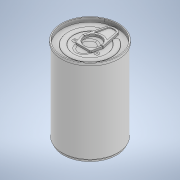
# Autodesk Inventor part: SoupCan
Saved by Autodesk Inventor 2020 (Build 240168000, 168)
## iProperties
Created: 2023-01-12
Part Number: SoupCan
Material: Generic
Document SubType Name: Modeling
Designer: legoo
Density: 1 g/cm^3
Appearance: Default
Author: legoo
Autodesk Inventor part; units mm, degrees
ref_plane "XZ Plane" through (0, 0, 0) normal (0, 1, 0) x (-1, 0, 0)
ref_plane "XY Plane" through (0, 0, 0) normal (0, 0, 1) x (1, 0, 0)
sketch "Sketch1" plane through (0, 0, 0) normal (0, 0, 1) x (1, 0, 0)
  line L0 (32.75, 4.0593) -> (32.75, 99.4351)
  line L1 (32.35, 97.4351) -> (0, 97.4351)
  line L2 (0, 97.4351) -> (0, 3.7133)
  line L3 (32.75, 99.4351) -> (33.55, 99.4351)
  line L4 (33.55, 99.4351) -> (33.55, 102.2351)
  line L5 (33.55, 102.2351) -> (32.35, 102.2351)
  line L6 (32.35, 102.2351) -> (32.35, 97.4351)
  line L7 (15, 3.7133) -> (0, 3.7133)
  arc A0 (15, 3.7133) -> (19.7851, 2.9089) centre (17.6851, 5.0514) ccw
  arc A1 (22.5851, 2.9089) -> (26.5659, 2.7142) centre (24.6851, 5.0514) ccw
  arc A2 (22.5851, 2.9089) -> (19.7851, 2.9089) centre (21.1851, 1.4807) ccw
  arc A3 (29.3384, 2.4576) -> (26.5659, 2.7142) centre (27.8198, 1.1561) ccw
  arc A4 (31.8792, 2.7098) -> (32.75, 4.0593) centre (30.8031, 4.3599) ccw
  arc A5 (31.2467, 0.7007) -> (31.8792, 2.7098) centre (28.3022, 2.7319) ccw
  arc A6 (29.9974, 0.7007) -> (31.2467, 0.7007) centre (30.622, 1.3024) ccw
  line L8 (29.3384, 2.4576) -> (29.9974, 0.7007)
  point P0 (0, 0)
  point P1 (30.622, 0.4351)
  dimension "d0" = 1.2
  dimension "d1" = 0.8
  dimension "d2" = 2.8
  dimension "d3" = 4.8
  dimension "d5" = 32.75
  dimension "d7" = 2
  dimension "d8" = 3
  dimension "d10" = 3
  dimension "d11" = 7
  dimension "d13" = 0
  dimension "d14" = 2
  dimension "d15" = 0
  dimension "d16" = 15
  dimension "d18" = 101.8
  dimension "d19" = 0.4351
  constraints: 18 end point, 16 point on circle, 7 centre point, 3 parallel, 3 tangent, 1 horizontal, 1 perpendicular
  measures "d0" distance of L4.end L5.end
  measures "d1" distance between parallel lines of L4 L0
  measures "d2" distance of L3.end L4.end
  measures "d3" distance between parallel lines of L1 L5
  measures "d5" distance between parallel lines of L2 L0
  measures "d7" radius of A2
  measures "d8" radius of A0
  measures "d10" radius of A1
  measures "d11" distance of A1.centre A0.centre
  measures "d13" vertical distance of A0.centre A1.centre
  measures "d14" radius of A3
  measures "d15" distance from line of point (0, 0) L2
  measures "d16" distance of L7.start L2.end
  measures "d18" distance from line of L5 point (30.622, 0.435)
  measures "d19" vertical distance of point (0, 0) point (30.622, 0.435)
revolve "Revolution1" add sketch "Sketch1" angle 360 about axis through (0, 97.4351, 0) along (0, -1, 0)
sketch "Sketch2" plane through (0, 97.4351, 0) normal (0, 1, 0) x (1, 0, 0)
  arc A0 (-12.675, 21.9537) -> (12.675, 21.9537) centre (0, 0) ccw
  arc A1 (-9.675, 16.7576) -> (9.675, 16.7576) centre (0, 0) ccw
  line L0 (0, 0) -> (-14.6692, 25.4078) construction
  line L1 (0, 0) -> (14.3618, 24.8753) construction
  circle A2 centre (0, 0) radius 32.35 construction
  circle A3 centre (0, 0) radius 22.35 construction
  arc A4 (-9.675, 16.7576) -> (-12.675, 21.9537) centre (-11.175, 19.3557) ccw
  arc A5 (12.675, 21.9537) -> (9.675, 16.7576) centre (11.175, 19.3557) ccw
  line L2 (0, 0) -> (0, 29.3384) construction
  circle A6 centre (0, 0) radius 29.3384 construction
  dimension "d20" = 6
  dimension "d21" = 7
  dimension "d22" = 3
  dimension "d23" = 60
  dimension "d48" = 30
  dimension "d53" = 0
  dimension "d54" = 0
  constraints: 10 point on circle, 6 end point, 5 centre point, 4 point on line, 3 coincident, 1 vertical, 2 other
  measures "d20" radial gap between concentric circles of A1 A0
  measures "d21" radial gap between concentric circles of A0 A2
  measures "d22" radial gap between concentric circles of A3 A0
  measures "d23" angle of L1 L0
  measures "d48" angle of L1 L2
  measures "d53" distance of point (0, 0) L1.start
  measures "d54" distance of point (0, 0) L1.start
extrude "Extrusion1" add sketch "Sketch2" along normal blind 0.25
chamfer "Chamfer1" distance 0.25 angle 45 4 edges at (0, 97.4351, 25.35) (-8.5769, 97.4351, -20.8557) (0, 97.4351, 19.35) (8.5769, 97.4351, -20.8557)
sketch "Sketch3" plane through (0, 97.4351, 0) normal (0, 1, 0) x (1, 0, 0)
  ellipse E0 centre (0, -4.1) end of major axis (0, 5.9) minor radius 7.5
  arc A0 (-9.55, 16.5411) -> (9.55, 16.5411) centre (0, 0) ccw construction
  point P0 (0, 0)
  point P1 (0, -19.1)
  point P2 (0, -14.1)
  dimension "d29" = 10
  dimension "d30" = 7.5
  dimension "d31" = 5
  constraints: 1 point on circle, 1 vertical alignment, 2 other
  measures "d31" distance of point (0, -14.1) point (0, -19.1)
extrude "Extrusion2" cut sketch "Sketch3" against normal blind 0.6
chamfer "Chamfer2" distance 0.6 distance2 2.5 1 edges at (0, 97.4351, 14.1) measured on face at (-7.3349, 97.0351, 6.1869)
sketch "Sketch4" plane through (0, 97.4351, 0) normal (0, 1, 0) x (1, 0, 0)
  circle A0 centre (-13, -4.85) radius 2.5
  circle A1 centre (13, -4.85) radius 2.5
  arc A2 (-9.675, 16.7576) -> (9.675, 16.7576) centre (0, 0) ccw construction
  point P0 (0, 0)
  point P1 (0, -19.35)
  dimension "d37" = 5
  dimension "d38" = 5
  dimension "d39" = 14.5
  dimension "d40" = 14.5
  dimension "d41" = 13
  dimension "d42" = 13
  constraints: 2 centre point, 1 point on circle
  measures "d37" diameter of A1
  measures "d38" diameter of A0
  measures "d39" vertical distance of point (0, -19.35) A0.centre
  measures "d40" vertical distance of point (0, -19.35) A1.centre
  measures "d41" horizontal distance of A0.centre point (0, 0)
  measures "d42" horizontal distance of point (0, 0) A1.centre
extrude "Extrusion3" add sketch "Sketch4" along normal blind 0.6
fillet "Fillet1" radius 2.5 2 edges at (10.5, 98.0351, 4.85) (-15.5, 98.0351, 4.85)
sketch "Sketch5" plane through (0, 97.4351, 0) normal (0, 1, 0) x (1, 0, 0)
  ellipse E0 centre (0, 25.85) end of major axis (-6.85, 25.85) minor radius 4 (6.85, 25.85) -> (-6.85, 25.85) ccw
  circle A0 centre (0, 0) radius 32.35 construction
  line L0 (6.85, 25.85) -> (11.7977, 3.6347)
  line L1 (-6.85, 25.85) -> (-11.7977, 3.6347)
  line L2 (11.7899, 3.1673) -> (9.0436, -7.4689)
  line L3 (-11.7899, 3.1673) -> (-9.0436, -7.4689)
  line L4 (-8.0754, -8.2189) -> (8.0754, -8.2189)
  arc A1 (-9.0436, -7.4689) -> (-8.0754, -8.2189) centre (-8.0754, -7.2189) ccw
  arc A2 (8.0754, -8.2189) -> (9.0436, -7.4689) centre (8.0754, -7.2189) ccw
  arc A3 (11.7899, 3.1673) -> (11.7977, 3.6347) centre (10.8217, 3.4173) ccw
  arc A4 (-11.7977, 3.6347) -> (-11.7899, 3.1673) centre (-10.8217, 3.4173) ccw
  point P0 (0, 32.35)
  point P1 (0, 29.85)
  point P2 (0, 29.85)
  point P3 (11.85, 3.4001)
  point P4 (-11.85, 3.4001)
  point P5 (8.85, -8.2189)
  point P6 (-8.85, -8.2189)
  dimension "d46" = 6.85
  dimension "d47" = 4
  dimension "d49" = 0
  dimension "d50" = 2.5
  dimension "d51" = 0
  dimension "d52" = 0
  dimension "d57" = 5
  dimension "d59" = 23
  dimension "d60" = 23
  dimension "d61" = 5
  dimension "d62" = 3
  dimension "d63" = 3
  dimension "d64" = 12
  dimension "d65" = 12
  dimension "d68" = 0
  dimension "d69" = 0
  dimension "d70" = 1
  constraints: 10 end point, 8 point on circle, 8 point on line, 8 tangent, 4 centre point, 3 equal radius, 1 coincident, 1 vertical alignment, 6 other
  measures "d49" horizontal distance of point (0, 0) point (0, 25.85)
  measures "d50" distance of point (0, 32.35) point (0, 29.85)
  measures "d51" horizontal distance of point (0, 0) point (0, 29.85)
  measures "d52" horizontal distance of point (0, 0) point (0, 32.35)
  measures "d57" horizontal distance of point (11.85, 3.4) L0.start
  measures "d59" distance of L0.start point (11.85, 3.4)
  measures "d60" distance of L1.start point (-11.85, 3.4)
  measures "d61" horizontal distance of point (-11.85, 3.4) L1.start
  measures "d62" horizontal distance of point (8.85, -8.219) point (11.85, 3.4)
  measures "d63" horizontal distance of point (-11.85, 3.4) point (-8.85, -8.219)
  measures "d64" distance of point (11.85, 3.4) point (8.85, -8.219)
  measures "d65" distance of point (-11.85, 3.4) point (-8.85, -8.219)
  measures "d68" vertical distance of point (0, 25.85) L0.start
  measures "d69" vertical distance of point (0, 25.85) L1.start
  measures "d70" radius of A1
extrude "Extrusion4" add sketch "Sketch5" along normal blind 2.6
ref_plane "Work Plane1" through (-12.7, 0, 0) normal (1, 0, 0) x (0, 1, 0)
sketch "Sketch6" plane through (-12.7, 0, 0) normal (1, 0, 0) x (0, 1, 0)
  line L0 (99.4351, 32.75) -> (99.4351, -32.75) projected
  line L1 (99.4351, -29.7539) -> (100.0351, -3.6347)
  line L2 (100.0351, -3.6347) -> (100.0351, -3.1673) projected
  line L3 (100.0351, -3.6347) -> (100.0351, -3.1673)
  line L4 (100.0351, -3.1673) -> (99.4351, 8.2189)
  line L5 (97.4351, 8.2189) -> (100.0351, 8.2189) projected
  line L6 (99.4351, 8.2189) -> (104.5755, 8.3468)
  line L7 (104.5755, 8.3468) -> (104.5755, -29.7539)
  line L8 (104.5755, -29.7539) -> (99.4351, -29.7539)
  point P0 (0, 0)
  constraints: 12 end point, 2 point on line, 1 perpendicular, 1 vertical
extrude "Extrusion5" cut sketch "Sketch6" along normal blind 25 contours L6 L7 L8 L1 L2 L4
sketch "Sketch7" plane through (0, 100.0351, 0) normal (0, 1, 0) x (1, 0, 0)
  line L0 (-11.7899, 3.1673) -> (11.7899, 3.1673) projected
  circle A0 centre (0, 3.1673) radius 9.25
  point P0 (0, 0)
  dimension "d78" = 18.5
  constraints: 1 centre point, 1 midpoint
  measures "d78" diameter of A0
extrude "Extrusion6" cut sketch "Sketch7" against normal up to surface (2.6 mm away)
fillet "Fillet2" radius 0.5 2 edges at (0, 99.8333, -12.4173) (0, 99.5476, 6.0827)
sketch "Sketch8" plane through (0, 100.0351, 0) normal (0, 1, 0) x (1, 0, 0)
  arc A0 (9.7393, 3.6347) -> (-9.7393, 3.6347) centre (0, 3.1788) ccw projected
  line L0 (11.7977, 3.6347) -> (9.7393, 3.6347) projected
  line L1 (6.85, 25.85) -> (11.7977, 3.6347) projected
  ellipse E0 centre (0, 25.85) end of major axis (-6.85, 25.85) minor radius 4 (6.85, 25.85) -> (1.4925, 29.7539) ccw projected
  line L2 (-1.4925, 29.7539) -> (1.4925, 29.7539) projected
  ellipse E1 centre (0, 25.85) end of major axis (-6.85, 25.85) minor radius 4 (-1.4925, 29.7539) -> (-6.85, 25.85) ccw projected
  line L3 (-11.7977, 3.6347) -> (-6.85, 25.85) projected
  line L4 (-9.7393, 3.6347) -> (-11.7977, 3.6347) projected
  line L5 (1.3563, 27.7539) -> (-1.3563, 27.7539)
  arc A1 (11.7412, 3.6347) -> (11.7234, 3.9683) centre (0, 3.1788) ccw
  line L6 (9.7487, 3.6347) -> (9.7366, 3.689)
  line L7 (7.6055, 13.2576) -> (4.8288, 25.7253)
  arc A2 (6.827, 12.742) -> (-6.827, 12.742) centre (0, 3.1788) ccw
  arc A3 (-11.7234, 3.9683) -> (-11.7412, 3.6347) centre (0, 3.1788) ccw
  line L8 (-4.8288, 25.7253) -> (-7.6055, 13.2576)
  line L9 (-9.7366, 3.689) -> (-9.7487, 3.6347)
  arc A4 (6.827, 12.742) -> (7.6055, 13.2576) centre (7.1175, 13.1489) ccw
  arc A5 (-7.6055, 13.2576) -> (-6.827, 12.742) centre (-7.1175, 13.1489) ccw
  spline S0 degree 5 poles (4.8287, 25.7253) (4.8473, 25.7837) (4.8599, 25.8452) (4.8521, 25.9084) (4.7769, 26.1544) (4.6074, 26.3574) (4.4736, 26.4956) (4.0346, 26.864) (3.5296, 27.1369) (3.1835, 27.2887) (2.6137, 27.4909) (2.0273, 27.6354) (1.8048, 27.6821) (1.5811, 27.7215) (1.3563, 27.7539) knots 0 0 0 0 0 0 0.071407 0.071407 0.071407 0.297158 0.297158 0.297158 0.735529 0.735529 0.735529 1 1 1 1 1 1
  spline S1 degree 5 poles (-1.3563, 27.7539) (-1.5811, 27.7215) (-1.8048, 27.6821) (-2.0273, 27.6354) (-2.6137, 27.4909) (-3.1835, 27.2887) (-3.5296, 27.1369) (-4.0346, 26.864) (-4.4736, 26.4956) (-4.6074, 26.3574) (-4.7769, 26.1544) (-4.8521, 25.9084) (-4.8599, 25.8452) (-4.8473, 25.7837) (-4.8287, 25.7253) knots 0 0 0 0 0 0 0.264471 0.264471 0.264471 0.702842 0.702842 0.702842 0.928593 0.928593 0.928593 1 1 1 1 1 1
  point P0 (0, 0)
  point P1 (7.9164, 11.8617)
  point P2 (-7.9164, 11.8617)
  dimension "d83" = 0.5
  constraints: 14 point on circle, 10 end point, 8 point on line, 5 centre point, 4 tangent, 2 parallel, 1 equal radius, 8 other
  measures "d83" radius of A4
extrude "Extrusion7" cut sketch "Sketch8" against normal blind 1.5 contours S0 L7 A4 A2 A5 L8 S1 L5
equation "\"d40\" = d39"
equation "\"d42\" = d41"
body "Solid1"
